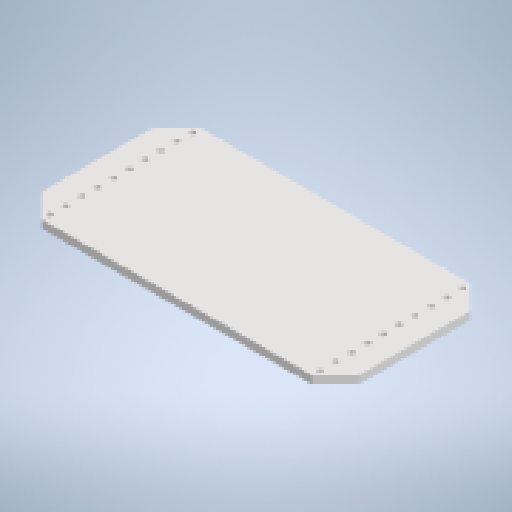
# Autodesk Inventor part: Chasis2
Saved by Autodesk Inventor 2024 (Build 280153000, 153)
## iProperties
Created: 2024-03-25
Part Number: Chasis2
Material: Generic
Document SubType Name: Modeling
Designer: JDAM
Density: 1 g/cm^3
Appearance: Default
Author: JDAM
Autodesk Inventor part; units mm, degrees
ref_plane "YZ Plane" through (0, 0, 0) normal (1, 0, 0) x (0, 1, 0)
ref_plane "XZ Plane" through (0, 0, 0) normal (0, 1, 0) x (-1, 0, 0)
ref_plane "XY Plane" through (0, 0, 0) normal (0, 0, 1) x (1, 0, 0)
sketch "Sketch1" plane through (0, 0, 0) normal (0, 1, 0) x (-1, 0, 0)
  line L0 (-100, 50) -> (100, 50)
  line L1 (100, 50) -> (100, -50)
  line L2 (100, -50) -> (-100, -50)
  line L3 (-100, -50) -> (-100, 50)
  line L4 (-100, 50) -> (100, -50) construction
  line L5 (100, 50) -> (-100, -50) construction
  point P0 (0, 0)
  dimension "d0" = 200
  dimension "d1" = 100
  constraints: 12 end point, 2 midpoint, 2 parallel, 1 horizontal, 1 perpendicular
  measures "d0" distance of L1.end L2.end
  measures "d1" distance of L0.end L1.end
extrude "Extrusion1" add sketch "Sketch1" along normal blind 5
chamfer "Chamfer1" distance 15 angle 45 4 edges at (100, 2.5, -50) (100, 2.5, 50) (-100, 2.5, 50) (-100, 2.5, -50)
sketch "Sketch2" plane through (0, 5, 0) normal (0, 1, 0) x (1, 0, 0)
  line L0 (-85, -50) -> (85, -50) projected
  line L1 (85, 50) -> (85, -50)
  line L2 (85, 0) -> (0, 0)
  line L3 (85, 50) -> (-85, 50) projected
  line L4 (85, 0) -> (75, 0)
  line L5 (75, 0) -> (75, 50)
  line L6 (85, -50) -> (85, -45)
  line L7 (85, -45) -> (87.1749, -45)
  dimension "d7" = 10
  dimension "d15" = 5
  constraints: 12 end point, 3 point on line, 2 horizontal, 1 midpoint, 1 perpendicular, 1 vertical
  measures "d7" distance of L2.start L4.end
  measures "d15" distance of L0.end L6.end
hole "Hole2" at (85, 5, 45) direction (0, -1, 0) diameter 3.5 depth 12
pattern_linear "Rectangular Pattern1" count 10 spacing 10 along (0, 0, -1) of "Hole2"
mirror "Mirror1" about plane through (0, 0, 0) normal (1, 0, 0) of "Hole2", "Rectangular Pattern1"
body "Solid1"
